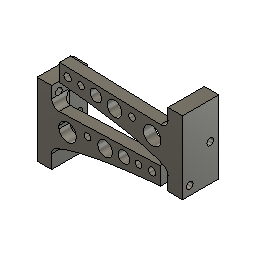
metal rack brackets v1 (Autodesk Fusion 360 design; units mm, degrees)
Autodesk Fusion 360 part; units mm, degrees
sketch "Sketch1" plane through (0, 0, 0) normal (0, 0, 1) x (1, 0, 0)
  line L0 (0, 0) -> (0, 25)
  line L1 (0, 25) -> (10, 25)
  line L2 (10, 25) -> (10, 0)
  line L3 (10, 0) -> (0, 0)
  line L4 (10, 0) -> (84.954312, 2.617462)
  line L5 (84.954312, 2.617462) -> (84.535518, 14.610152)
  line L6 (84.535518, 14.610152) -> (10, 12.007315)
  line L7 (0, 0) -> (0, -25)
  line L8 (0, -25) -> (10, -25)
  line L9 (10, -25) -> (10, 0)
  spline S0 degree 5 poles (84.954312, 2.617462) (81.970417, 2.340419) (76.098134, 1.765867) (67.576229, 0.842646) (56.796201, -0.513137) (44.372117, -2.43306) (33.134471, -4.60721) (23.263712, -7.074254) (14.959292, -9.87693) (8.40383, -13.054369) (3.691636, -16.626779) (1.358685, -19.792582) (0.383274, -22.33285) (0.071357, -24.098865) (0, -25) knots 0 0 0 0 0 0 0.1 0.2 0.3 0.4 0.5 0.6 0.7 0.8 0.9 1 1 1 1 1 1
  point P0 (10, -12.5)
  dimension "d1" = 25
  dimension "d2" = 75
  dimension "d3" = 182
  dimension "d4" = 12
  dimension "d5" = 25
  dimension "d6" = 12.5
  constraint coincident L0.start L3.end
  constraint vertical L0
  constraint perpendicular L0 L1
  constraint perpendicular L1 L2
  constraint perpendicular L0 L3
  constraint perpendicular L4 L5
  constraint perpendicular L5 L6
  constraint perpendicular L3 L7
  constraint perpendicular L2 L8
  constraint parallel L2 L9
  constraint coincident L9 P0
  measures "d1" distance of L0.start L0.end
  measures "d5" distance of L0.start L7.end
  measures "d6" distance of L8.end P0
extrude "Extrude1" add sketch "Sketch1" along normal mid plane 15 contours L2 L4 L5 L6 | L4 L9 S0 picked at (34.984771, 4.874926) picked at (20.244867, -4.547872) makes body 1
extrude "Extrude2" add sketch "Sketch1" along normal mid plane 50 contours L0 L1 L2 L3 | L3 L7 L9 S0 | L8 L9 S0 picked at (3.333333, 12.335772) picked at (6.666667, -4.166667) picked at (9.054796, -17.2487) bodies 1
sketch "Sketch2" plane through (10, 0, 0) normal (1, 0, 0) x (0, 0, -1)
  line L0 (25, 25) -> (-25, 25)
  line L1 (-25, 25) -> (-25, -25)
  line L2 (-25, -25) -> (25, -25)
  line L3 (25, -25) -> (25, 25)
  line L4 (7.5, 12.007315) -> (7.5, -12.5)
  line L5 (7.5, -12.5) -> (-7.5, -12.5)
  line L6 (-7.5, -12.5) -> (-7.5, 12.007315)
  line L7 (-7.5, 12.007315) -> (7.5, 12.007315)
  circle A0 centre (5, 19) radius 2.25
  circle A1 centre (-19, 0) radius 2.25
  circle A2 centre (-5, -19) radius 2.25
  circle A3 centre (19, 0) radius 2.25
  line L8 (0, 38.233351) -> (0, -31.858375) construction
  dimension "d11" = 4.5
  dimension "d16" = 6
  dimension "d17" = 20
  dimension "d22" = 20
  constraint perpendicular L5 L8
  measures "d11" diameter of A0
  measures "d16" distance of L0 A0.centre
  measures "d17" distance of L3 A0.centre
  measures "d22" distance of L1 A2.centre
extrude "Extrude3" cut sketch "Sketch2" against normal blind 20 contours A0 | A1 | A2 | A3 picked at (4.53416, 20.320067) picked at (-19.384849, 0.714862) picked at (-4.380321, -19.597769) picked at (17.556526, 0.610516) bodies 1
fillet "Fillet1" radius 5 4 edges at (10, -0.246343, 7.5) (10, -12.5, 0) (10, -0.246343, -7.5) (10, 12.007315, 0) on bodies 1
sketch "Sketch3" plane through (0, 0, -7.5) normal (0, 0, -1) x (-1, 0, 0)
  line L0 (-15, -10.13167) -> (-15, 12.184966)
  arc A0 (-15.174497, 12.188012) -> (-15, 12.184966) centre (-15, 17.184966) ccw
  line L1 (-15.174497, 12.188012) -> (-84.535518, 14.610152)
  line L2 (-84.535518, 14.610152) -> (-84.954312, 2.617462)
  spline S0 degree 5 poles (-84.954312, 2.617462) (-81.970417, 2.340419) (-76.098134, 1.765867) (-67.576229, 0.842646) (-56.796201, -0.513137) (-44.372117, -2.43306) (-33.134471, -4.60721) (-25.13187, -6.607337) (-19.833729, -8.270544) (-16.62726, -9.465523) (-15.078658, -10.099321) (-15, -10.13167) knots 0 0 0 0 0 0 0.1 0.2 0.3 0.4 0.5 0.6 0.60536907 0.60536907 0.60536907 0.60536907 0.60536907 0.60536907
  line L3 (-84.744915, 8.613807) -> (-10.715526, 6.028644) construction
  circle A1 centre (-69.744915, 8.089996) radius 2.25
  circle A2 centre (-34.744915, 6.867769) radius 2.25
  circle A3 centre (-46.740666, 5.857279) radius 5
  circle A4 centre (-20.915548, 2.674706) radius 6
  circle A5 centre (-79.049694, 8.414926) radius 2.5
  circle A6 centre (-59.652821, 7.321226) radius 4
  dimension "d24" = 4.5
  dimension "d25" = 4.5
  dimension "d26" = 15
  dimension "d27" = 50
  dimension "d30" = 10
  dimension "d31" = 12
  dimension "d32" = 5
  dimension "d33" = 8
  constraint perpendicular L2 L3
  measures "d24" diameter of A1
  measures "d25" diameter of A2
  measures "d30" diameter of A3
  measures "d31" diameter of A4
  measures "d32" diameter of A5
  measures "d33" diameter of A6
extrude "Extrude4" cut sketch "Sketch3" against normal blind 40 contours L0 A4 | A1 | A2 | A3 | A5 | A6 picked at (-19.134296, 2.941513) picked at (-70.319647, 8.932973) picked at (-35.018921, 7.632005) picked at (-48.24228, 7.740245) picked at (-79.489638, 9.535885) picked at (-60.882574, 7.122503) bodies 1
ref_plane "WorkPlane1" through (0, 0, 0) normal (0, 0, 1) x (1, 0, 0)
split "Split1" by plane through (0, 0, 0) normal (0, 0, 1) bodies 1 makes body 2 at (0, 17.364822, 14.392661)
move_body "Move1" bodies 2 to x (-1, 0, 0) y (0, 1, 0) z (0, 0, -1) at (100, 27, -0.011903)
